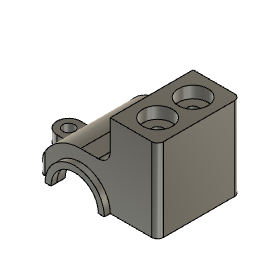
drawing_24 (Autodesk Fusion 360 design; units mm, degrees)
Autodesk Fusion 360 part; units mm, degrees
sketch "Sketch1" plane through (0, 0, 0) normal (0, 0, 1) x (1, 0, 0)
  line L0 (20, 35) -> (-20, 35)
  line L1 (-20, 35) -> (-20, -35)
  line L2 (-20, -35) -> (20, -35)
  line L3 (20, -35) -> (20, 35)
  line L4 (20, 35) -> (-20, -35) construction
  line L5 (-20, 35) -> (20, -35) construction
  dimension "d1" = 40
  dimension "d2" = 70
  constraint horizontal L0
  constraint perpendicular L0 L1
  constraint parallel L0 L2
  constraint parallel L1 L3
  constraint coincident L4 origin
  constraint coincident L5 origin
  measures "d1" distance of L1.end L2.end
  measures "d2" distance of L0.end L1.end
extrude "Extrude1" add sketch "Sketch1" along normal blind 70 makes body 1
sketch "Sketch2" plane through (0, 0, 70) normal (0, 0, 1) x (-1, 0, 0)
  line L0 (-20, 35) -> (-20, -35)
  line L1 (-20, -35) -> (20, -35)
  line L2 (20, -35) -> (20, 35)
  line L3 (20, 35) -> (-20, 35)
  line L4 (-12.7745, -35) -> (-15, -35)
  line L5 (-20, -30) -> (-20, -29)
  line L6 (-20, 30) -> (-20, 31)
  line L7 (-15, 35) -> (-15, 35)
  arc A0 (-20, -30) -> (-15, -35) centre (-15, -30) ccw
  arc A1 (-15, 35) -> (-20, 30) centre (-15, 30) ccw
  dimension "d5" = 5
  dimension "d6" = 5
  constraint coincident L1 L4.start
  constraint perpendicular L0 L4
  constraint coincident L0 L5.end
  constraint perpendicular L4 L5
  constraint coincident L0 L6.end
  constraint perpendicular L3 L6
  constraint coincident L3 L7.start
  constraint tangent L5 A0
  constraint tangent L4 A0
  constraint tangent L6 A1
  measures "d5" radius of A0
  measures "d6" radius of A1
extrude "Extrude2" cut sketch "Sketch2" against normal blind 133 contours L0 L3 L6 A1 | L0 L1 A0 bodies 1
sketch "Sketch3" plane through (0, 0, 70) normal (0, 0, 1) x (-1, 0, 0)
  arc A0 (-20, -30) -> (-15, -35) centre (-15, -30) ccw
  line L0 (-15, -35) -> (20, -35)
  line L1 (20, -35) -> (20, 35)
  line L2 (20, 35) -> (-15, 35)
  arc A1 (-15, 35) -> (-20, 30) centre (-15, 30) ccw
  line L3 (-20, 30) -> (-20, -30)
  line L4 (-20, 0) -> (-20, -15) construction
  line L5 (-20, 0) -> (-20, 15) construction
  line L6 (0, -15) -> (0, 15) construction
  circle A2 centre (0, -15) radius 5
  circle A3 centre (0, 15) radius 5
  point P0 (-20, 0)
  dimension "d9" = 15
  dimension "d10" = 15
  dimension "d11" = 10
  dimension "d12" = 10
  constraint midpoint L3 P0
  constraint coincident P0 L4.start
  constraint parallel L3 L4
  constraint parallel L3 L5
  constraint parallel L3 L6
  constraint coincident L6.start A2.centre
  constraint coincident L6.end A3.centre
  measures "d9" distance of P0 L4.end
  measures "d10" distance of P0 L5.end
  measures "d11" diameter of A2
  measures "d12" diameter of A3
extrude "Extrude3" cut sketch "Sketch3" against normal blind 100 contours A2 | A3 bodies 1
sketch "Sketch4" plane through (0, 0, 70) normal (0, 0, 1) x (-1, 0, 0)
  circle A0 centre (0, -15) radius 5
  circle A1 centre (0, 15) radius 5
  arc A2 (-20, -30) -> (-15, -35) centre (-15, -30) ccw
  line L0 (-15, -35) -> (20, -35)
  line L1 (20, -35) -> (20, 35)
  line L2 (20, 35) -> (-15, 35)
  arc A3 (-15, 35) -> (-20, 30) centre (-15, 30) ccw
  line L3 (-20, 30) -> (-20, -30)
  circle A4 centre (0, -15) radius 12.5
  circle A5 centre (0, 15) radius 12.5
  dimension "d15" = 25
  dimension "d16" = 25
  constraint concentric A0 A4
  constraint concentric A1 A5
  measures "d15" diameter of A4
  measures "d16" diameter of A5
extrude "Extrude4" cut sketch "Sketch4" against normal blind 10 contours A4 | A5 bodies 1
sketch "Sketch5" plane through (0, -35, 0) normal (0, -1, 0) x (1, 0, 0)
  line L0 (15, 0) -> (15, 70)
  line L1 (15, 70) -> (-20, 70)
  line L2 (-20, 70) -> (-20, 0)
  line L3 (-20, 0) -> (15, 0)
  line L4 (15, 0) -> (20, 0)
  line L5 (20, 0) -> (20, 70)
  line L6 (20, 70) -> (15, 70)
  line L7 (15, 70) -> (15, 0)
  line L8 (-20, 0) -> (0, 0) construction
  line L9 (0, 0) -> (-45, 0) construction
  circle A0 centre (-45, 0) radius 35
  line L10 (-80, 0) -> (-20, 0)
  dimension "d19" = 45
  dimension "d20" = 70
  constraint coincident L2.end L3.start
  constraint coincident L8.end L9.start
  constraint perpendicular L0 L9
  constraint coincident L9.end A0.centre
  constraint coincident A0 L10.start
  constraint perpendicular L2 L10
  measures "d19" distance of L8.end L9.end
  measures "d20" diameter of A0
extrude "Extrude5" add sketch "Sketch5" against normal blind 70 contours L2 L3 A0 | L2 A0 L10 bodies 1
sketch "Sketch6" plane through (0, -35, 0) normal (0, -1, 0) x (1, 0, 0)
  line L0 (-80, 0) -> (15, 0)
  line L1 (15, 0) -> (15, 70)
  line L2 (15, 70) -> (-20, 70)
  line L3 (-20, 70) -> (-20, 24.4949)
  arc A0 (-20, 24.4949) -> (-80, 0) centre (-45, 0) ccw
sketch "Sketch7" plane through (0, 0, 0) normal (0, 0, -1) x (1, 0, 0)
  line L0 (-80, -35) -> (15, -35)
  arc A0 (15, -35) -> (20, -30) centre (15, -30) ccw
  line L1 (20, -30) -> (20, 30)
  arc A1 (20, 30) -> (15, 35) centre (15, 30) ccw
  line L2 (15, 35) -> (-80, 35)
  line L3 (-80, 35) -> (-80, -35)
  circle A2 centre (0, -15) radius 5
  circle A3 centre (0, 15) radius 5
  line L4 (-75, 35) -> (-70, 35)
  line L5 (-80, 30) -> (-80, 25)
  line L6 (-80, -30) -> (-80, -27.174)
  line L7 (-75, -35) -> (-70, -35)
  arc A4 (-75, 35) -> (-80, 30) centre (-75, 30) ccw
  arc A5 (-80, -30) -> (-75, -35) centre (-75, -30) ccw
  dimension "d23" = 5
  dimension "d24" = 5
  constraint coincident L2 L4.end
  constraint coincident L3 L5.end
  constraint perpendicular L2 L5
  constraint coincident L3 L6.end
  constraint perpendicular L0 L6
  constraint coincident L0 L7.end
  constraint perpendicular L3 L7
  constraint tangent L4 A4
  constraint tangent L5 A4
  constraint tangent L6 A5
  constraint tangent L7 A5
  measures "d23" radius of A4
  measures "d24" radius of A5
extrude "Extrude6" cut sketch "Sketch7" against normal blind 100 contours L0 L3 A5 | L2 L3 A4 bodies 1
sketch "Sketch8" plane through (0, -35, 0) normal (0, -1, 0) x (1, 0, 0)
  line L0 (-80, 0) -> (-45, 0) construction
  circle A0 centre (-45, 0) radius 20
  dimension "d27" = 40
  constraint horizontal L0
  constraint coincident L0.end A0.centre
  measures "d27" diameter of A0
extrude "Extrude7" cut sketch "Sketch8" against normal blind 110 bodies 1
sketch "Sketch9" plane through (0, -35, 0) normal (0, -1, 0) x (1, 0, 0)
  circle A0 centre (-45, 0) radius 25
  line L0 (-70, 0) -> (-20, 0)
  circle A1 centre (-45, 0) radius 20
  dimension "d30" = 50
  dimension "d31" = 40
  constraint coincident A0 L0.start
  constraint coincident A0 L0.end
  constraint horizontal L0
  constraint concentric A0 A1
  measures "d30" diameter of A0
  measures "d31" diameter of A1
extrude "Extrude8" add sketch "Sketch9" along normal blind 5 and the other way blind 75 contours A0 L0 A1 picked at (-68.2403, 1.242) bodies 1
sketch "Sketch10" plane through (-20, 0, 0) normal (-1, 0, 0) x (0, -1, 0)
  line L0 (-35, 24.4949) -> (35, 24.4949)
  line L1 (35, 24.4949) -> (35, 70)
  line L2 (35, 70) -> (-35, 70)
  line L3 (-35, 70) -> (-35, 24.4949)
  spline S0 degree 3 poles (30, 0) (30.5549, 1.468) (31.1345, 2.9997) (32.2614, 6.1023) (32.8087, 7.6732) (33.7767, 10.7745) (34.1983, 12.305) (34.8087, 15.2592) (35, 16.6825) (35, 18.0278) knots 0 0 0 0 0.470823 0.470823 0.941647 0.941647 1.41247 1.41247 1.883293 1.883293 1.883293 1.883293
  line L4 (35, 18.0278) -> (35, 35)
  line L5 (35, 24.4949) -> (-35, 24.4949)
  line L6 (-35, 35) -> (-35, 18.0278)
  spline S1 degree 3 poles (-35, 18.0278) (-35, 16.6825) (-34.8087, 15.2592) (-34.1983, 12.305) (-33.7767, 10.7745) (-32.8087, 7.6732) (-32.2614, 6.1023) (-31.1345, 2.9997) (-30.5549, 1.468) (-30, 0) knots 3.924114 3.924114 3.924114 3.924114 4.394938 4.394938 4.865761 4.865761 5.336584 5.336584 5.807408 5.807408 5.807408 5.807408
  line L7 (-30, 0) -> (30, 0)
  line L8 (-35, 35) -> (35, 35)
  line L9 (35, 35) -> (35, 24.4949)
  line L10 (35, 24.4949) -> (-35, 24.4949)
  line L11 (-35, 24.4949) -> (-35, 35)
  constraint horizontal L8
  constraint vertical L9
  constraint horizontal L10
  constraint vertical L11
  constraint coincident L0.end L1.start
  constraint coincident L6.start L8.start
extrude "Extrude9" add sketch "Sketch10" along normal blind 25 contours L0 L1 L3 L4 L5 L6 L8 L9 L10 L11 bodies 1
sketch "Sketch11" plane through (0, -35, 0) normal (0, -1, 0) x (1, 0, 0)
  arc A0 (-20, 0) -> (-70, 0) centre (-45, 0) ccw
  line L0 (-20, 0) -> (15, 0)
  line L1 (15, 0) -> (15, 70)
  line L2 (15, 70) -> (-20, 70)
  line L3 (-20, 70) -> (-20, 35)
  line L4 (-20, 35) -> (-45, 35)
  arc A1 (-45, 35) -> (-75, 18.0278) centre (-45, 0) ccw
  line L5 (-75, 18.0278) -> (-75, 0)
  line L6 (-75, 0) -> (-70, 0)
  line L7 (-20, 45) -> (-20, 47)
  line L8 (-30, 35) -> (-28, 35)
  arc A2 (-30, 35) -> (-20, 45) centre (-30, 45) ccw
  dimension "d38" = 10
  constraint coincident L3 L7.end
  constraint perpendicular L4 L7
  constraint coincident L4 L8.end
  constraint perpendicular L3 L8
  constraint tangent L7 A2
  constraint tangent L8 A2
  measures "d38" radius of A2
extrude "Extrude10" add sketch "Sketch11" against normal blind 70 contours L3 L4 L8 A2 bodies 1
sketch "Sketch12" plane through (0, 0, 0) normal (0, 0, -1) x (1, 0, 0)
  line L0 (-20, -35) -> (15, -35)
  arc A0 (15, -35) -> (20, -30) centre (15, -30) ccw
  line L1 (20, -30) -> (20, 30)
  arc A1 (20, 30) -> (15, 35) centre (15, 30) ccw
  line L2 (15, 35) -> (-20, 35)
  line L3 (-20, 35) -> (-20, 40)
  line L4 (-20, 40) -> (-25, 40)
  line L5 (-25, 40) -> (-25, 35)
  line L6 (-25, 35) -> (-25, -35)
  line L7 (-25, -35) -> (-25, -40)
  line L8 (-25, -40) -> (-20, -40)
  line L9 (-20, -40) -> (-20, -35)
  circle A2 centre (0, 15) radius 5
  circle A3 centre (0, -15) radius 5
  line L10 (15, -35) -> (-20, -35)
  line L11 (-75, -35) -> (-70, -35)
  line L12 (-20, 35) -> (15, 35)
  line L13 (-70, 35) -> (-75, 35)
  line L14 (-70, 35) -> (-70, 40)
  line L15 (-20, 40) -> (-70, 40)
  line L16 (-20, 40) -> (-20, 35)
  line L17 (-20, -35) -> (-20, -40)
  line L18 (-70, -40) -> (-20, -40)
  line L19 (-70, -40) -> (-70, -35)
  line L20 (-80, 30) -> (-80, -30)
  spline S0 degree 3 poles (-80, 30) (-80, 30.5549) (-79.9063, 31.1345) (-79.4994, 32.2614) (-79.1863, 32.8087) (-78.3391, 33.7767) (-77.805, 34.1983) (-76.5395, 34.8087) (-75.8084, 35) (-75, 35) knots 0 0 0 0 0.470823 0.470823 0.941647 0.941647 1.41247 1.41247 1.883293 1.883293 1.883293 1.883293
  spline S1 degree 3 poles (-75, -35) (-75.8084, -35) (-76.5395, -34.8087) (-77.805, -34.1983) (-78.3391, -33.7767) (-79.1863, -32.8087) (-79.4994, -32.2614) (-79.9063, -31.1345) (-80, -30.5549) (-80, -30) knots 3.924114 3.924114 3.924114 3.924114 4.394938 4.394938 4.865761 4.865761 5.336584 5.336584 5.807408 5.807408 5.807408 5.807408
  circle A4 centre (0, 15) radius 5
  circle A5 centre (0, -15) radius 5
  arc A6 (15, -35) -> (20, -30) centre (15, -30) ccw
  arc A7 (20, 30) -> (15, 35) centre (15, 30) ccw
  line L21 (20, 30) -> (20, -30)
  circle A8 centre (0, -15) radius 5
  circle A9 centre (0, -15) radius 12.5
  circle A10 centre (0, 15) radius 5
  circle A11 centre (0, 15) radius 12.5
  line L22 (20, 20) -> (13, 20) construction
  line L23 (20, 0) -> (20, 28) construction
  line L24 (-45, 40) -> (-45, -40) construction
  line L25 (13, 28) -> (-45, 28)
  line L26 (-45, 28) -> (-45, -28)
  line L27 (-45, -28) -> (13, -28)
  line L28 (13, -28) -> (13, 28)
  point P0 (-45, 40)
  point P1 (-45, 12.8704)
  dimension "d41" = 7
  dimension "d42" = 28
  dimension "d43" = 56
  constraint coincident L1 L22.start
  constraint perpendicular L1 L22
  constraint midpoint L21 L23.start
  constraint parallel L1 L23
  constraint midpoint L15 P0
  constraint coincident P0 L24.start
  constraint midpoint L18 L24.end
  constraint horizontal L25
  constraint vertical L26
  constraint horizontal L27
  constraint vertical L28
  constraint coincident L24 L26.end
  measures "d41" distance of L22.start L22.end
  measures "d42" distance of L23.start L23.end
  measures "d43" distance of L25.start L27.end
extrude "Extrude11" add sketch "Sketch12" against normal blind 28 separate body contours L6 L25 L26 L27 | L6 L25 L27 L28 makes body 2
sketch "Sketch13" plane through (0, -28, 0) normal (0, -1, 0) x (1, 0, 0)
  line L0 (-45, 0) -> (13, 0)
  line L1 (13, 0) -> (13, 28)
  line L2 (13, 28) -> (-45, 28)
  line L3 (-45, 28) -> (-45, 0)
  circle A0 centre (-45, 0) radius 28
  line L4 (-45, 0) -> (-73, 0)
  dimension "d46" = 56
  constraint coincident L0.start L3.end
  constraint coincident A0 L4.end
  constraint perpendicular L3 L4
  measures "d46" diameter of A0
extrude "Extrude12" add sketch "Sketch13" against normal blind 56 contours L3 A0 L4 bodies 2
sketch "Sketch14" plane through (0, -28, 0) normal (0, -1, 0) x (1, 0, 0)
  line L0 (-73, 0) -> (13, 0)
  line L1 (13, 0) -> (13, 28)
  line L2 (13, 28) -> (-45, 28)
  arc A0 (-45, 28) -> (-73, 0) centre (-45, 0) ccw
  line L3 (13, 23) -> (13, 22.7078)
  line L4 (8, 28) -> (7.9644, 28)
  arc A1 (13, 23) -> (8, 28) centre (8, 23) ccw
  dimension "d49" = 5
  constraint coincident L1 L3.end
  constraint perpendicular L2 L3
  constraint coincident L2 L4.end
  constraint perpendicular L1 L4
  constraint tangent L4 A1
  constraint tangent L3 A1
  measures "d49" radius of A1
extrude "Extrude13" cut sketch "Sketch14" against normal blind 85 contours L1 L2 A1 bodies 2
extrude "Extrude14" cut 1 faces at (-35, -28, 9.3333) along direction (0, 1, 0) blind 56 on bodies 2 bodies 1 2
sketch "Sketch15" plane through (0, -35, 0) normal (0, -1, 0) x (1, 0, 0)
  arc A0 (-20, 0) -> (-70, 0) centre (-45, 0) ccw
  line L0 (-20, 0) -> (15, 0)
  line L1 (15, 0) -> (15, 70)
  line L2 (15, 70) -> (-20, 70)
  line L3 (-20, 70) -> (-20, 45)
  arc A1 (-30, 35) -> (-20, 45) centre (-30, 45) ccw
  line L4 (-30, 35) -> (-45, 35)
  arc A2 (-45, 35) -> (-75, 18.0278) centre (-45, 0) ccw
  line L5 (-75, 18.0278) -> (-75, 0)
  line L6 (-75, 0) -> (-70, 0)
  spline S0 degree 3 poles (-80, 0) (-80, 1.468) (-79.9063, 2.9997) (-79.4994, 6.1023) (-79.1863, 7.6732) (-78.3391, 10.7745) (-77.805, 12.305) (-76.5395, 15.2592) (-75.8084, 16.6825) (-75, 18.0278) knots 0 0 0 0 0.470823 0.470823 0.941647 0.941647 1.41247 1.41247 1.883293 1.883293 1.883293 1.883293
  spline S1 degree 3 poles (-80, 0) (-80, 1.468) (-79.9063, 2.9997) (-79.4994, 6.1023) (-79.1863, 7.6732) (-78.3391, 10.7745) (-77.805, 12.305) (-76.5395, 15.2592) (-75.8084, 16.6825) (-75, 18.0278) knots 0 0 0 0 0.470823 0.470823 0.941647 0.941647 1.41247 1.41247 1.883293 1.883293 1.883293 1.883293
  line L7 (-80, 0) -> (-75, 0)
  line L8 (-75, 0) -> (-75, 18.0278)
  line L9 (15, 0) -> (20, 0)
  line L10 (20, 0) -> (20, 70)
  line L11 (20, 70) -> (15, 70)
  line L12 (15, 70) -> (15, 0)
  line L13 (20, 0) -> (-90, 0) construction
  dimension "d54" = 110
  constraint coincident L9.end L10.start
  constraint perpendicular L1 L13
  measures "d54" distance of L9.end L13.end
sketch "Sketch16" plane through (0, 0, 0) normal (0, 0, 1) x (1, 0, 0)
  circle A0 centre (0, 15) radius 5
  circle A1 centre (0, -15) radius 5
  line L0 (-70, -40) -> (-65, -40)
  line L1 (-70, -35) -> (-70, -40)
  line L2 (-75, -35) -> (-70, -35)
  arc A2 (-80, -30) -> (-75, -35) centre (-75, -30) ccw
  line L3 (-80, -30) -> (-80, 30)
  arc A3 (-75, 35) -> (-80, 30) centre (-75, 30) ccw
  line L4 (-70, 35) -> (-75, 35)
  line L5 (-70, 40) -> (-70, 35)
  line L6 (-65, 40) -> (-70, 40)
  line L7 (15, 35) -> (-20, 35)
  line L8 (-20, -35) -> (15, -35)
  line L9 (-20, -40) -> (-20, -35)
  line L10 (-20, 35) -> (-20, 40)
  line L11 (-25, 40) -> (-65, 40)
  line L12 (-65, -40) -> (-25, -40)
  line L13 (-20, 40) -> (-25, 40)
  line L14 (-25, -40) -> (-20, -40)
  arc A4 (20, 30) -> (15, 35) centre (15, 30) ccw
  line L15 (20, -30) -> (20, 30)
  arc A5 (15, -35) -> (20, -30) centre (15, -30) ccw
  line L16 (20, 0) -> (-74, 0) construction
  line L17 (-90, -10) -> (-74, -10)
  line L18 (-74, -10) -> (-74, 10)
  line L19 (-74, 10) -> (-90, 10)
  arc A6 (-90, 10) -> (-90, -10) centre (-90, 0) ccw
  dimension "d55" = 110
  dimension "d56" = 20
  constraint midpoint L15 L16.start
  constraint perpendicular L15 L16
  constraint tangent L17 A6
  constraint perpendicular L3 L17
  constraint perpendicular L16 L18
  constraint tangent L19 A6
  constraint coincident L18 L16.end
  measures "d55" distance of L16.start A6.centre
  measures "d56" diameter of A6
extrude "Extrude15" add sketch "Sketch16" along normal blind 10 contours L3 L17 L19 A6 | L3 L17 L18 L19 bodies 1 2
sketch "Sketch17" plane through (0, 0, 10) normal (0, 0, 1) x (-1, 0, 0)
  line L0 (78.541, 10) -> (78.541, -10)
  line L1 (78.541, -10) -> (90, -10)
  arc A0 (90, -10) -> (90, 10) centre (90, 0) ccw
  line L2 (90, 10) -> (78.541, 10)
  circle A1 centre (90, 0) radius 5
  dimension "d59" = 10
  constraint concentric A0 A1
  measures "d59" diameter of A1
extrude "Extrude16" cut sketch "Sketch17" against normal blind 28 contours A1 bodies 1
equation "d42 = ( 56 / 2 ) * 1 mm"
